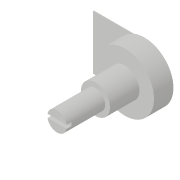
# Autodesk Inventor part: pot.0001
Saved by Autodesk Inventor 2018 (Build 220112000, 112)
## iProperties
Created: 2019-04-23
Part Number: pot.0001
Material: Generic
Document SubType Name: Modeling
Designer: amink
Density: 1 g/cm^3
Appearance: Default
Author: amink
Autodesk Inventor part; units mm, degrees
ref_plane "YZ Plane" through (0, 0, 0) normal (1, 0, 0) x (0, 1, 0)
ref_plane "XZ Plane" through (0, 0, 0) normal (0, 1, 0) x (-1, 0, 0)
ref_plane "XY Plane" through (0, 0, 0) normal (0, 0, 1) x (1, 0, 0)
sketch "Sketch1" plane through (0, 0, 0) normal (0, 0, 1) x (1, 0, 0)
  circle A0 centre (0, 0) radius 9.525
  dimension "d0" = 19.05
  constraints: 1 centre point, 1 coincident
  measures "d0" diameter of A0
extrude "Extrusion1" add sketch "Sketch1" along normal blind 6.35
sketch "Sketch2" plane through (0, 0, 6.35) normal (0, 0, 1) x (1, 0, 0)
  circle A0 centre (0, 0) radius 4.7625
  dimension "d3" = 9.525
  constraints: 1 centre point, 1 coincident
  measures "d3" diameter of A0
extrude "Extrusion2" add sketch "Sketch2" along normal blind 9.652
sketch "Sketch3" plane through (0, 0, 16.002) normal (0, 0, 1) x (1, 0, 0)
  circle A0 centre (0, 0) radius 3.175
  dimension "d6" = 6.35
  constraints: 1 centre point, 1 coincident
  measures "d6" diameter of A0
extrude "Extrusion3" add sketch "Sketch3" along normal blind 12.573
sketch "Sketch4" plane through (0, 0, 28.575) normal (0, 0, 1) x (1, 0, 0)
  line L0 (-6.35, 0.5969) -> (6.35, 0.5969)
  line L1 (6.35, 0.5969) -> (6.35, -0.5969)
  line L2 (6.35, -0.5969) -> (-6.35, -0.5969)
  line L3 (-6.35, -0.5969) -> (-6.35, 0.5969)
  point P0 (0, 0)
  dimension "d9" = 1.1938
  dimension "d10" = 12.7
  dimension "d11" = 6.35
  dimension "d12" = 0.5969
  constraints: 8 end point, 2 parallel, 1 horizontal, 1 perpendicular
  measures "d9" distance between parallel lines of L2 L0
  measures "d10" distance of L0.start L0.end
  measures "d11" distance from line of point (0, 0) L3
  measures "d12" distance from line of point (0, 0) L0
extrude "Extrusion4" cut sketch "Sketch4" against normal blind 1.6002
sketch "Sketch5" plane through (0, 0, 0) normal (0, 0, -1) x (-1, 0, 0)
  circle A0 centre (0, 0) radius 9.525 projected
  line L0 (3.4196, 8.89) -> (16.51, 8.89)
  line L1 (16.51, 8.89) -> (16.51, -8.89)
  line L2 (16.51, -8.89) -> (3.4196, -8.89)
  line L3 (0, -8.89) -> (0, 9.525)
  line L4 (3.4196, -8.89) -> (0, -8.89)
  line L5 (3.4196, 8.89) -> (0, 8.89)
  dimension "d15" = 16.51
  dimension "d18" = 17.78
  dimension "d19" = 8.89
  constraints: 12 end point, 2 horizontal, 2 parallel, 2 perpendicular, 2 point on line, 1 vertical alignment, 1 other
  measures "d15" distance between parallel lines of L3 L1
  measures "d18" distance between parallel lines of L0 L2
  measures "d19" distance from line of point (0, 0) L0
extrude "Extrusion5" add sketch "Sketch5" against normal blind 0.254
equation "\"d11\" = 0.5 * d10"
equation "\"d12\" = 0.5 * d9"
equation "\"d19\" = 0.5 * d18"
body "Solid1"
